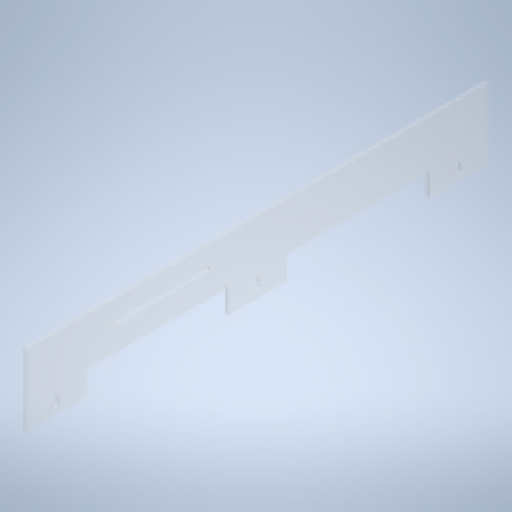
# Autodesk Inventor part: 라즈베리파이보관_옆판
Saved by Autodesk Inventor 2024 (Build 280153000, 153)
## iProperties
Created: 2024-04-10
Part Number: 라즈베리파이보관_옆판
Material: PMMA 플라스틱
Document SubType Name: Modeling
Designer: kkamin5
Density: 1.188 g/cm^3
Appearance: 폴리카보네이트 - 선명
Mass: 110.484 g
Surface Area: 415.2 cm^2
Volume: 93 cm^3
Author: kkamin5
Autodesk Inventor part; units mm, degrees
ref_plane "YZ Plane" through (0, 0, 0) normal (1, 0, 0) x (0, 1, 0)
ref_plane "XZ Plane" through (0, 0, 0) normal (0, 1, 0) x (-1, 0, 0)
ref_plane "XY Plane" through (0, 0, 0) normal (0, 0, 1) x (1, 0, 0)
sketch "스케치1" plane through (0, 0, 0) normal (1, 0, 0) x (0, 1, 0)
  line L0 (30, 195) -> (-30, 195)
  line L1 (-30, 195) -> (-30, -195)
  line L2 (-30, -195) -> (30, -195)
  line L3 (30, -195) -> (30, 195)
  point P0 (0, 0)
  dimension "d0" = 60
  dimension "d1" = 390
  dimension "d2" = 30
  dimension "d3" = 195
  constraints: 8 end point, 2 parallel, 1 horizontal, 1 perpendicular
  measures "d0" distance of L2.end L1.end
  measures "d1" distance of L1.end L0.end
  measures "d2" distance from line of point (0, 0) L3
  measures "d3" distance from line of point (0, 0) L0
extrude "돌출1" add sketch "스케치1" along normal blind 3
sketch "스케치2" plane through (3, 0, 0) normal (1, 0, 0) x (0, 0, -1)
  line L0 (-195, -30) -> (195, -30) projected
  line L1 (-145, -30) -> (-25, -30)
  line L2 (-25, -30) -> (-25, -10)
  line L3 (-25, -10) -> (-145, -10)
  line L4 (-145, -10) -> (-145, -30)
  line L5 (-195, 30) -> (-195, -30) projected
  line L6 (0, 0) -> (0, -66.648) construction
  line L7 (25, -10) -> (145, -10)
  line L8 (145, -10) -> (145, -30)
  line L9 (145, -30) -> (25, -30)
  line L10 (25, -30) -> (25, -10)
  line L11 (195, -30) -> (195, 30) projected
  dimension "d6" = 20
  dimension "d7" = 50
  dimension "d8" = 25
  dimension "d9" = 50
  dimension "d10" = 25
  dimension "d11" = 20
  constraints: 18 end point, 4 parallel, 2 horizontal, 2 perpendicular, 2 point on line, 1 vertical
  measures "d6" distance of L2.end L1.end
  measures "d7" distance between parallel lines of L5 L4
  measures "d8" distance from line of L6.start L2
  measures "d9" distance between parallel lines of L11 L8
  measures "d10" distance between parallel lines of L6 L10
  measures "d11" distance between parallel lines of L0 L7
extrude "돌출2" cut sketch "스케치2" against normal through all
sketch "스케치3" plane through (3, 0, 0) normal (1, 0, 0) x (0, 0, -1)
  line L0 (-170, 132.4891) -> (-170, -92.5)
  line L1 (0, 133.9107) -> (0, -104.4082)
  line L2 (170, 113.5044) -> (170, -115.928)
  line L3 (195, -30) -> (195, 30) projected
  line L4 (-195, 30) -> (-195, -30) projected
  line L5 (-170, -22) -> (-170, -18) construction
  line L6 (-168, -22) -> (-168, -18)
  line L7 (-172, -18) -> (-172, -22)
  arc A0 (-172, -22) -> (-168, -22) centre (-170, -22) ccw
  arc A1 (-168, -18) -> (-172, -18) centre (-170, -18) ccw
  line L8 (0, -22) -> (0, -18) construction
  line L9 (2, -22) -> (2, -18)
  line L10 (-2, -18) -> (-2, -22)
  arc A2 (-2, -22) -> (2, -22) centre (0, -22) ccw
  arc A3 (2, -18) -> (-2, -18) centre (0, -18) ccw
  line L11 (170, -22) -> (170, -18) construction
  line L12 (172, -22) -> (172, -18)
  line L13 (168, -18) -> (168, -22)
  arc A4 (168, -22) -> (172, -22) centre (170, -22) ccw
  arc A5 (172, -18) -> (168, -18) centre (170, -18) ccw
  line L14 (145, -30) -> (195, -30) projected
  line L15 (-25, -30) -> (25, -30) projected
  line L16 (-195, -30) -> (-145, -30) projected
  line L17 (-120, 10) -> (-40, 10)
  line L18 (-40, 10) -> (-40, 13)
  line L19 (-40, 13) -> (-120, 13)
  line L20 (-120, 13) -> (-120, 10)
  point P0 (0, 0)
  point P1 (-170, -20)
  point P2 (0, -20)
  point P3 (170, -20)
  dimension "d14" = 25
  dimension "d15" = 25
  dimension "d16" = 0
  dimension "d17" = 4
  dimension "d18" = 4
  dimension "d19" = 4
  dimension "d20" = 4
  dimension "d21" = 4
  dimension "d22" = 4
  dimension "d23" = 10
  dimension "d24" = 10
  dimension "d25" = 10
  dimension "d36" = 80
  dimension "d37" = 3
  dimension "d38" = 75
  dimension "d39" = 10
  constraints: 38 end point, 12 point on circle, 12 tangent, 6 centre point, 6 point on line, 5 parallel, 3 midpoint, 3 vertical, 1 horizontal, 1 perpendicular
  measures "d14" distance between parallel lines of L3 L2
  measures "d15" distance between parallel lines of L4 L0
  measures "d16" distance from line of L1 point (0, 0)
  measures "d17" distance of L5.start L5.end
  measures "d18" diameter of A1
  measures "d19" distance of L8.start L8.end
  measures "d20" diameter of A3
  measures "d21" distance of L11.start L11.end
  measures "d22" diameter of A5
  measures "d23" distance from line of L14 point (170, -20)
  measures "d24" distance from line of L15 point (0, -20)
  measures "d25" distance from line of L16 point (-170, -20)
  measures "d36" distance of L19.end L18.end
  measures "d37" distance of L18.end L17.end
  measures "d38" distance from line of L4 L17.start
  measures "d39" distance from line of point (0, 0) L17
extrude "돌출3" cut sketch "스케치3" against normal blind 10
equation "\"d3\" = 0.5 * d1"
equation "\"d6\" = d11"
equation "\"d10\" = d8"
